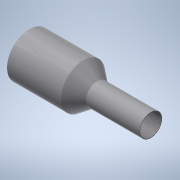
# Autodesk Inventor part: Tubo tolba
Saved by Autodesk Inventor 2020 (Build 240168000, 168)
## iProperties
Created: 2020-02-16
Part Number: Tubo tolba
Material: Steel, Mild, Welded
Document SubType Name: Modeling
Designer: PabloGod
Density: 7.85 g/cm^3
Appearance: Weld - Steel Mild
Author: PabloGod
Autodesk Inventor part; units mm, degrees
ref_plane "YZ Plane" through (0, 0, 0) normal (1, 0, 0) x (0, 1, 0)
ref_plane "XZ Plane" through (0, 0, 0) normal (0, 1, 0) x (-1, 0, 0)
ref_plane "XY Plane" through (0, 0, 0) normal (0, 0, 1) x (1, 0, 0)
sketch "Boceto1" plane through (0, 0, 0) normal (1, 0, 0) x (0, 1, 0)
  circle A0 centre (0, 0) radius 60
  circle A1 centre (0, 0) radius 62
  line L0 (0, 0) -> (1013.9731, 0) construction
  dimension "d0" = 120
  dimension "d1" = 124
  constraints: 2 centre point, 2 coincident, 2 end point, 1 horizontal
  measures "d0" diameter of A0
  measures "d1" diameter of A1
extrude "Extrusión1" add sketch "Boceto1" along normal blind 150
ref_plane "Plano de trabajo1" through (190, 0, 0) normal (1, 0, 0) x (0, 0, -1)
sketch "Boceto4" plane through (190, 0, 0) normal (1, 0, 0) x (0, 0, -1)
  circle A0 centre (0, 0) radius 30
  circle A1 centre (0, 0) radius 31.5
  dimension "d6" = 60
  dimension "d7" = 63
  constraints: 2 centre point, 2 coincident
  measures "d6" diameter of A0
  measures "d7" diameter of A1
extrude "Extrusión2" add sketch "Boceto4" along normal blind 150
loft "Solevación1" add section 1 edges at (190, 0, 31.5) section 2 edges at (150, -62, 0) section 3 edges at (190, 0, 30)
